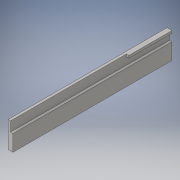
# Autodesk Inventor part: Base Runner Side Right
Saved by Autodesk Inventor 2016 (Build 200138000, 138)
## iProperties
Created: 2017-11-04
Part Number: Base Runner Side Right
Material: Generic
Document SubType Name: Modeling
Designer: mathaetaes
Density: 1 g/cm^3
Appearance: Default
Author: mathaetaes
Autodesk Inventor part; units mm, degrees
ref_plane "YZ Plane" through (0, 0, 0) normal (1, 0, 0) x (0, 1, 0)
ref_plane "XZ Plane" through (0, 0, 0) normal (0, 1, 0) x (-1, 0, 0)
ref_plane "XY Plane" through (0, 0, 0) normal (0, 0, 1) x (1, 0, 0)
sketch "Sketch1" plane through (0, 0, 0) normal (1, 0, 0) x (0, 1, 0)
  line L0 (64.7557, 308.0174) -> (-36.8443, 308.0174)
  line L1 (-36.8443, 308.0174) -> (-36.8443, -314.2826)
  line L2 (-36.8443, -314.2826) -> (64.7557, -314.2826)
  line L3 (64.7557, -314.2826) -> (64.7557, 308.0174)
  dimension "d2" = 622.3
  dimension "d3" = 101.6
  constraints: 8 end point, 2 parallel, 1 horizontal, 1 perpendicular
  measures "d2" distance of L0.end L1.end
  measures "d3" distance of L1.end L2.end
extrude "Board" add sketch "Sketch1" along normal blind 19.05
sketch "Sketch8" plane through (19.05, 0, 0) normal (1, 0, 0) x (0, 0, -1)
  line L0 (-308.0174, 55.2307) -> (314.2826, 55.2307)
  line L1 (314.2826, 55.2307) -> (314.2826, 45.7057)
  line L2 (314.2826, 45.7057) -> (-308.0174, 45.7057)
  line L3 (-308.0174, 45.7057) -> (-308.0174, 55.2307)
  line L4 (-308.0174, 64.7557) -> (-308.0174, -36.8443) projected
  line L5 (314.2826, -36.8443) -> (314.2826, 64.7557) projected
  line L6 (314.2826, 64.7557) -> (-308.0174, 64.7557) projected
  point P0 (0, 0)
  dimension "d22" = 9.525
  dimension "d23" = 9.525
  constraints: 8 end point, 2 collinear, 2 parallel, 1 horizontal, 1 perpendicular
  measures "d22" distance of L0.end L1.end
  measures "d23" distance between parallel lines of L6 L0
extrude "Lenghtwise Dado for Base" cut sketch "Sketch8" against normal blind 9.525 contours L0 L1 L2 L3
sketch "Sketch 9" plane through (0, 64.7557, 308.0174) normal (0, 1, 0) x (1, 0, 0)
  line L0 (19.05, 0) -> (9.525, 0)
  line L1 (9.525, 0) -> (9.525, 454.025)
  line L2 (9.525, 454.025) -> (19.05, 454.025)
  line L3 (19.05, 454.025) -> (19.05, 0)
  line L4 (19.05, 622.3) -> (19.05, 0) projected
  line L5 (0, 622.3) -> (19.05, 622.3) projected
  line L6 (0, 0) -> (19.05, 0) projected
  point P0 (0, 308.0174)
  dimension "d26" = 454.025
  dimension "d27" = 9.525
  constraints: 8 end point, 2 collinear, 2 parallel, 1 horizontal, 1 perpendicular
  measures "d26" distance of L2.end L0.start
  measures "d27" distance of L1.end L2.end
extrude "Lengthwise stop dado for Sides" cut sketch "Sketch 9" against normal blind 9.525
sketch "Sketch12" plane through (19.05, 0, 0) normal (1, 0, 0) x (0, 0, -1)
  line L0 (-308.0174, 26.6557) -> (314.2826, 26.6557)
  line L1 (314.2826, 26.6557) -> (314.2826, 45.7057)
  line L2 (314.2826, 45.7057) -> (-308.0174, 45.7057)
  line L3 (-308.0174, 45.7057) -> (-308.0174, 26.6557)
  line L4 (314.2826, 45.7057) -> (-308.0174, 45.7057) projected
  line L5 (-308.0174, 45.7057) -> (-308.0174, -36.8443) projected
  line L6 (314.2826, -36.8443) -> (314.2826, 45.7057) projected
  point P0 (0, 0)
  dimension "d30" = 19.05
  constraints: 8 end point, 3 collinear, 2 parallel, 1 horizontal, 1 perpendicular
  measures "d30" distance between parallel lines of L2 L0
extrude "Lenghtwise full dado for base" cut sketch "Sketch12" against normal blind 9.525
body "Solid1"
